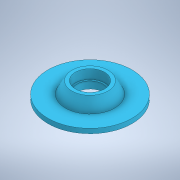
# Autodesk Inventor part: base reaction wheel
Saved by Autodesk Inventor 2022.2 (Build 262287000, 287)
## iProperties
Created: 2021-07-29
Part Number: base reaction wheel
Material: ABS Plastic
Document SubType Name: Modeling
Designer: samlo
Density: 1.06 g/cm^3
Appearance: Turquoise
Author: samlo
Autodesk Inventor part; units mm, degrees
ref_plane "YZ Plane" through (0, 0, 0) normal (1, 0, 0) x (0, 1, 0)
ref_plane "XZ Plane" through (0, 0, 0) normal (0, 1, 0) x (-1, 0, 0)
ref_plane "XY Plane" through (0, 0, 0) normal (0, 0, 1) x (1, 0, 0)
sketch "Sketch2" plane through (0, 0, 0) normal (0, 0, 1) x (1, 0, 0)
  line L0 (11, 0) -> (36, 0)
  line L1 (36, 0) -> (36, 4)
  line L2 (36, 4) -> (21, 4)
  line L3 (21, 4) -> (15.5, 14)
  line L4 (15.5, 14) -> (12.5, 14)
  line L5 (12.5, 14) -> (12.5, 6)
  line L6 (12.5, 6) -> (11, 6)
  line L7 (11, 6) -> (11, 0)
  line L8 (0, -2.8) -> (0, 16.8) projected
  point P0 (0, 0)
  dimension "d0" = 12.5
  dimension "d1" = 1.5
  dimension "d2" = 3
  dimension "d3" = 25
  dimension "d4" = 6
  dimension "d5" = 8
  dimension "d6" = 0
  dimension "d7" = 4
  dimension "d8" = 15
  constraints: 16 end point, 4 perpendicular, 2 horizontal, 1 parallel
  measures "d0" distance from line of L5 point (0, 0)
  measures "d1" distance of L5.end L6.end
  measures "d2" distance of L3.end L4.end
  measures "d3" distance of L0.start L0.end
  measures "d4" distance of L6.end L0.start
  measures "d5" distance of L4.end L5.end
  measures "d6" distance from line of point (0, 0) L0
  measures "d7" distance of L0.end L1.end
  measures "d8" distance of L1.end L2.end
revolve "Revolution1" add sketch "Sketch2" angle 360 about axis through (0, -10, 0) along (0, 1, 0)
body "Solid1"
